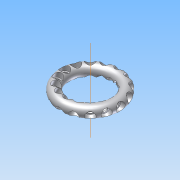
# Autodesk Inventor part: wheel
Saved by Autodesk Inventor 2012 (Build 160160000, 160)
## iProperties
Created: 2020-01-11
Part Number: wheel
Material: Default
Document SubType Name: Modeling
Designer: windows
Density: 1 g/cm^3
Mass: 34.9295 g
Surface Area: 256.992 cm^2
Volume: 34.9295 cm^3
Author: windows
Autodesk Inventor part; units mm, degrees
sketch "basic-frame" plane through (0, 0, 0) normal (0, 0, 1) x (1, 0, 0)
  line L0 (44.492, -8.85) -> (37.7185, -25.2027)
  line L1 (37.7185, -25.2027) -> (25.2027, -37.7185)
  line L2 (25.2027, -37.7185) -> (8.85, -44.492)
  line L3 (8.85, -44.492) -> (-8.85, -44.492)
  line L4 (-8.85, -44.492) -> (-25.2027, -37.7185)
  line L5 (-25.2027, -37.7185) -> (-37.7185, -25.2027)
  line L6 (-37.7185, -25.2027) -> (-44.492, -8.85)
  line L7 (-44.492, -8.85) -> (-44.492, 8.85)
  line L8 (-44.492, 8.85) -> (-37.7185, 25.2027)
  line L9 (-37.7185, 25.2027) -> (-25.2027, 37.7185)
  line L10 (-25.2027, 37.7185) -> (-8.85, 44.492)
  line L11 (-8.85, 44.492) -> (8.85, 44.492)
  line L12 (8.85, 44.492) -> (25.2027, 37.7185)
  line L13 (25.2027, 37.7185) -> (37.7185, 25.2027)
  line L14 (37.7185, 25.2027) -> (44.492, 8.85)
  line L15 (-73.9845, 0) -> (73.9845, 0) projected
  line L16 (44.492, 8.85) -> (44.492, -8.85)
  circle A0 centre (-44.492, 0) radius 7.6 construction
  circle A1 centre (-41.1052, -17.0263) radius 7.6 construction
  circle A2 centre (-31.4606, -31.4606) radius 7.6 construction
  circle A3 centre (-17.0263, -41.1052) radius 7.6 construction
  circle A4 centre (0, -44.492) radius 7.6 construction
  circle A5 centre (17.0263, -41.1052) radius 7.6 construction
  circle A6 centre (31.4606, -31.4606) radius 7.6 construction
  circle A7 centre (41.1052, -17.0263) radius 7.6 construction
  circle A8 centre (44.492, 0) radius 7.6 construction
  circle A9 centre (41.1052, 17.0263) radius 7.6 construction
  circle A10 centre (31.4606, 31.4606) radius 7.6 construction
  circle A11 centre (17.0263, 41.1052) radius 7.6 construction
  circle A12 centre (0, 44.492) radius 7.6 construction
  circle A13 centre (-17.0263, 41.1052) radius 7.6 construction
  circle A14 centre (-31.4606, 31.4606) radius 7.6 construction
  circle A15 centre (-41.1052, 17.0263) radius 7.6 construction
  circle A16 centre (-31.4606, 31.4606) radius 9.7599
  line L17 (-25.1935, 23.9786) -> (-37.7276, 38.9425)
  point P0 (0, 0)
  point P1 (0, 0)
  dimension "model_size" = 17.7
  dimension "d1" = 90.7272
  dimension "d106" = 15.2
  dimension "d109" = 360
  constraints: 34 end point, 17 centre point, 2 coincident, 2 midpoint, 2 point on circle, 2 point on line, 1 perpendicular, 1 tangent, 64 other
  measures "model_size" distance of L6.end L7.end
  measures "d1" distance of L0.start L7.end
  measures "d106" diameter of A0
ref_plane "plane-0" through (-44.492, -8.85, 0) normal (0, 0, 1) x (0, 1, 0)
sketch "circle-0" plane through (-44.492, -8.85, 0) normal (0, 0, 1) x (0, 1, 0)
  circle A0 centre (8.85, 0) radius 8.85
  line L0 (0, 0) -> (17.7, 0) projected
  circle A1 centre (8.85, 0) radius 7.6
  circle A2 centre (8.85, 0) radius 5
  point P0 (8.85, -44.492)
  dimension "model_de" = 15.2
  dimension "model_di" = 10
  constraints: 3 centre point, 2 coincident, 2 point on circle, 1 midpoint
  measures "model_de" diameter of A1
  measures "model_di" diameter of A2
ref_plane "plane-1" through (-37.7185, -25.2027, 0) normal (0.1802, 0.0747, 0.9808) x (-0.3827, 0.9239, 0)
sketch "circle-1" plane through (-37.7185, -25.2027, 0) normal (0.1802, 0.0747, 0.9808) x (-0.3827, 0.9239, 0)
  circle A0 centre (8.85, 0) radius 8.85
  line L0 (0, 0) -> (17.7, 0) projected
  circle A1 centre (8.85, 0) radius 5
  circle A2 centre (8.85, 0) radius 7.6
  point P0 (8.85, -43.6371)
  dimension "d76" = 10
  dimension "d77" = 15.2
  constraints: 3 centre point, 2 coincident, 2 point on circle, 1 midpoint
  measures "d76" diameter of A1
  measures "d77" diameter of A2
ref_plane "plane-2" through (-25.2027, -37.7185, 0) normal (0.2706, 0.2706, 0.9239) x (-0.7071, 0.7071, 0)
sketch "circle-2" plane through (-25.2027, -37.7185, 0) normal (0.2706, 0.2706, 0.9239) x (-0.7071, 0.7071, 0)
  line L0 (0, 0) -> (17.7, 0) projected
  circle A0 centre (8.85, 0) radius 8.85
  circle A1 centre (8.85, 0) radius 7.6
  circle A2 centre (8.85, 0) radius 5
  point P0 (8.85, -41.1052)
  dimension "d78" = 15.2
  dimension "d79" = 10
  constraints: 3 centre point, 2 coincident, 2 point on circle, 1 midpoint
  measures "d78" diameter of A1
  measures "d79" diameter of A2
ref_plane "plane-3" through (-8.85, -44.492, 0) normal (0.2126, 0.5133, 0.8315) x (-0.9239, 0.3827, 0)
sketch "circle-3" plane through (-8.85, -44.492, 0) normal (0.2126, 0.5133, 0.8315) x (-0.9239, 0.3827, 0)
  line L0 (0, 0) -> (17.7, 0) projected
  circle A0 centre (8.85, 0) radius 8.85
  circle A1 centre (8.85, 0) radius 7.6
  circle A2 centre (8.85, 0) radius 5
  point P0 (8.85, -36.9937)
  dimension "d80" = 15.2
  dimension "d81" = 10
  constraints: 3 coincident, 2 centre point, 1 horizontal alignment, 1 midpoint, 2 other
  measures "d80" diameter of A1
  measures "d81" diameter of A2
ref_plane "plane-4" through (8.85, -44.492, 0) normal (0, 0.7071, 0.7071) x (-1, 0, 0)
sketch "circle-4" plane through (8.85, -44.492, 0) normal (0, 0.7071, 0.7071) x (-1, 0, 0)
  circle A0 centre (8.85, 0) radius 8.85
  line L0 (0, 0) -> (17.7, 0) projected
  circle A1 centre (8.85, 0) radius 5
  circle A2 centre (8.85, 0) radius 7.6
  point P0 (8.85, -31.4606)
  dimension "d82" = 10
  dimension "d83" = 15.2
  constraints: 3 centre point, 2 coincident, 2 point on circle, 1 midpoint
  measures "d82" diameter of A1
  measures "d83" diameter of A2
ref_plane "plane-5" through (25.2027, -37.7185, 0) normal (-0.3182, 0.7682, 0.5556) x (-0.9239, -0.3827, 0)
sketch "circle-5" plane through (25.2027, -37.7185, 0) normal (-0.3182, 0.7682, 0.5556) x (-0.9239, -0.3827, 0)
  line L0 (0, 0) -> (17.7, 0) projected
  circle A0 centre (8.85, 0) radius 8.85
  circle A1 centre (8.85, 0) radius 7.6
  circle A2 centre (8.85, 0) radius 5
  point P0 (8.85, -24.7184)
  dimension "d84" = 15.2
  dimension "d85" = 10
  constraints: 3 centre point, 2 coincident, 2 point on circle, 1 midpoint
  measures "d84" diameter of A1
  measures "d85" diameter of A2
ref_plane "plane-6" through (37.7185, -25.2027, 0) normal (-0.6533, 0.6533, 0.3827) x (-0.7071, -0.7071, 0)
sketch "circle-6" plane through (37.7185, -25.2027, 0) normal (-0.6533, 0.6533, 0.3827) x (-0.7071, -0.7071, 0)
  circle A0 centre (8.85, 0) radius 8.85
  line L0 (0, 0) -> (17.7, 0) projected
  circle A1 centre (8.85, 0) radius 7.6
  circle A2 centre (8.85, 0) radius 5
  point P0 (8.85, -17.0263)
  dimension "d86" = 15.2
  dimension "d87" = 10
  constraints: 3 centre point, 2 coincident, 2 point on circle, 1 midpoint
  measures "d86" diameter of A1
  measures "d87" diameter of A2
ref_plane "plane-7" through (44.492, -8.85, 0) normal (-0.9061, 0.3753, 0.1951) x (-0.3827, -0.9239, 0)
sketch "circle-7" plane through (44.492, -8.85, 0) normal (-0.9061, 0.3753, 0.1951) x (-0.3827, -0.9239, 0)
  line L0 (0, 0) -> (17.7, 0) projected
  circle A0 centre (8.85, 0) radius 8.85
  circle A1 centre (8.85, 0) radius 7.6
  circle A2 centre (8.85, 0) radius 5
  point P0 (8.85, -8.6799)
  dimension "d88" = 15.2
  dimension "d89" = 10
  constraints: 3 centre point, 2 coincident, 2 point on circle, 1 midpoint
  measures "d88" diameter of A1
  measures "d89" diameter of A2
ref_plane "plane-8" through (44.492, 8.85, 0) normal (-1, 0, 0) x (0, -1, 0)
sketch "circle-8" plane through (44.492, 8.85, 0) normal (-1, 0, 0) x (0, -1, 0)
  circle A0 centre (8.85, 0) radius 8.85
  line L0 (0, 0) -> (17.7, 0) projected
  circle A1 centre (8.85, 0) radius 7.6
  circle A2 centre (8.85, 0) radius 5
  point P0 (8.85, 0)
  dimension "d90" = 15.2
  dimension "d91" = 10
  constraints: 3 centre point, 2 coincident, 2 point on circle, 1 midpoint
  measures "d90" diameter of A1
  measures "d91" diameter of A2
ref_plane "plane-9" through (37.7185, 25.2027, 0) normal (-0.9061, -0.3753, -0.1951) x (0.3827, -0.9239, 0)
sketch "circle-9" plane through (37.7185, 25.2027, 0) normal (-0.9061, -0.3753, -0.1951) x (0.3827, -0.9239, 0)
  circle A0 centre (8.85, 0) radius 8.85
  line L0 (0, 0) -> (17.7, 0) projected
  circle A1 centre (8.85, 0) radius 7.6
  circle A2 centre (8.85, 0) radius 5
  point P0 (8.85, 8.6799)
  dimension "d92" = 15.2
  dimension "d93" = 10
  constraints: 3 centre point, 2 coincident, 2 point on circle, 1 midpoint
  measures "d92" diameter of A1
  measures "d93" diameter of A2
ref_plane "plane-10" through (25.2027, 37.7185, 0) normal (-0.6533, -0.6533, -0.3827) x (0.7071, -0.7071, 0)
sketch "circle-10" plane through (25.2027, 37.7185, 0) normal (-0.6533, -0.6533, -0.3827) x (0.7071, -0.7071, 0)
  circle A0 centre (8.85, 0) radius 8.85
  line L0 (0, 0) -> (17.7, 0) projected
  circle A1 centre (8.85, 0) radius 7.6
  circle A2 centre (8.85, 0) radius 5
  point P0 (8.85, 17.0263)
  dimension "d94" = 15.2
  dimension "d95" = 10
  constraints: 3 centre point, 2 coincident, 2 point on circle, 1 midpoint
  measures "d94" diameter of A1
  measures "d95" diameter of A2
ref_plane "plane-11" through (8.85, 44.492, 0) normal (-0.3182, -0.7682, -0.5556) x (0.9239, -0.3827, 0)
sketch "circle-11" plane through (8.85, 44.492, 0) normal (-0.3182, -0.7682, -0.5556) x (0.9239, -0.3827, 0)
  circle A0 centre (8.85, 0) radius 8.85
  line L0 (0, 0) -> (17.7, 0) projected
  circle A1 centre (8.85, 0) radius 7.6
  circle A2 centre (8.85, 0) radius 5
  point P0 (8.85, 24.7184)
  dimension "d96" = 15.2
  dimension "d97" = 10
  constraints: 3 centre point, 2 coincident, 2 point on circle, 1 midpoint
  measures "d96" diameter of A1
  measures "d97" diameter of A2
ref_plane "plane-12" through (-8.85, 44.492, 0) normal (0, -0.7071, -0.7071) x (1, 0, 0)
sketch "circle-12" plane through (-8.85, 44.492, 0) normal (0, -0.7071, -0.7071) x (1, 0, 0)
  circle A0 centre (8.85, 0) radius 8.85
  line L0 (0, 0) -> (17.7, 0) projected
  circle A1 centre (8.85, 0) radius 7.6
  circle A2 centre (8.85, 0) radius 5
  point P0 (8.85, 31.4606)
  dimension "d98" = 15.2
  dimension "d99" = 10
  constraints: 3 centre point, 2 coincident, 2 point on circle, 1 midpoint
  measures "d98" diameter of A1
  measures "d99" diameter of A2
ref_plane "plane-13" through (-25.2027, 37.7185, 0) normal (0.2126, -0.5133, -0.8315) x (0.9239, 0.3827, 0)
sketch "circle-13" plane through (-25.2027, 37.7185, 0) normal (0.2126, -0.5133, -0.8315) x (0.9239, 0.3827, 0)
  circle A0 centre (8.85, 0) radius 8.85
  line L0 (0, 0) -> (17.7, 0) projected
  circle A1 centre (8.85, 0) radius 7.6
  circle A2 centre (8.85, 0) radius 5
  point P0 (8.85, 36.9937)
  dimension "d100" = 15.2
  dimension "d101" = 10
  constraints: 3 centre point, 2 coincident, 2 point on circle, 1 midpoint
  measures "d100" diameter of A1
  measures "d101" diameter of A2
ref_plane "plane-14" through (-37.7185, 25.2027, 0) normal (0.2706, -0.2706, -0.9239) x (0.7071, 0.7071, 0)
sketch "circle-14" plane through (-37.7185, 25.2027, 0) normal (0.2706, -0.2706, -0.9239) x (0.7071, 0.7071, 0)
  circle A0 centre (8.85, 0) radius 8.85
  line L0 (0, 0) -> (17.7, 0) projected
  circle A1 centre (8.85, 0) radius 7.6
  circle A2 centre (8.85, 0) radius 5
  point P0 (8.85, 41.1052)
  dimension "d102" = 15.2
  dimension "d103" = 10
  constraints: 3 centre point, 2 coincident, 2 point on circle, 1 midpoint
  measures "d102" diameter of A1
  measures "d103" diameter of A2
ref_plane "plane-15" through (-44.492, 8.85, 0) normal (0.1802, -0.0747, -0.9808) x (0.3827, 0.9239, 0)
sketch "circle-15" plane through (-44.492, 8.85, 0) normal (0.1802, -0.0747, -0.9808) x (0.3827, 0.9239, 0)
  line L0 (0, 0) -> (17.7, 0) projected
  circle A0 centre (8.85, 0) radius 8.85
  circle A1 centre (8.85, 0) radius 7.6
  circle A2 centre (8.85, 0) radius 5
  point P0 (8.85, 43.6371)
  dimension "d104" = 15.2
  dimension "d105" = 10
  constraints: 3 centre point, 2 coincident, 2 point on circle, 1 midpoint
  measures "d104" diameter of A1
  measures "d105" diameter of A2
ref_plane "工作平面17" through (-31.4606, 31.4606, 0) normal (0, 0, 1) x (1, 0, 0)
ref_plane "工作平面18" through (-31.4606, 31.4606, 0) normal (0.7071, 0.7071, 0) x (0, 0, 1)
sketch "草图22" plane through (-31.4606, 31.4606, 0) normal (0.7071, 0.7071, 0) x (0, 0, 1)
  line L0 (0, -9.7599) -> (0, 9.7599) projected
  line L1 (-14.0758, 0) -> (14.0758, 0) projected
  circle A0 centre (0, 0) radius 9.7599
  line L2 (-14.0758, 44.492) -> (14.0758, 44.492) projected
  point P0 (0, 44.492)
  constraints: 2 midpoint, 1 vertical alignment, 2 other
revolve "tire" add sketch "草图22" angle 360 about axis through (0, 0, -10) along (0, 0, 1)
extrude "hole0" cut sketch "circle-0" along normal through all both and the other way through all contours A1 L0 A2 | L0 A2 A1 | A2 L0 | L0 A2
extrude "support0" add sketch "circle-0" along normal mid plane 2 contours A1 L0 A2 | L0 A2 A1
extrude "hole1" cut sketch "circle-1" along normal through all both and the other way through all contours A2 L0 A1 | L0 A1 A2 | A1 L0 | L0 A1
extrude "support1" add sketch "circle-1" along normal mid plane 2 contours A2 L0 A1 | L0 A1 A2
extrude "hole2" cut sketch "circle-2" along normal through all both and the other way through all contours A2 L0 A1 | A2 L0 | L0 A2 | L0 A1 A2
extrude "support2" add sketch "circle-2" along normal mid plane 2 contours A2 L0 A1 | L0 A1 A2
extrude "hole3" cut sketch "circle-3" along normal through all both and the other way through all contours A2 L0 A1 | A2 L0 | L0 A2 | L0 A1 A2
extrude "support3" add sketch "circle-3" along normal mid plane 2 contours A2 L0 A1 | L0 A1 A2
extrude "hole4" cut sketch "circle-4" along normal through all both and the other way through all contours A2 L0 A1 | L0 A1 A2 | A1 L0 | L0 A1
extrude "support4" add sketch "circle-4" along normal mid plane 2 contours A2 L0 A1 | L0 A1 A2
extrude "hole5" cut sketch "circle-5" along normal through all both and the other way through all contours A2 L0 A1 | A2 L0 | L0 A2 | L0 A1 A2
extrude "support5" add sketch "circle-5" along normal mid plane 2 contours A2 L0 A1 | L0 A1 A2
extrude "hole6" cut sketch "circle-6" along normal through all both and the other way through all contours A1 L0 A2 | L0 A2 A1 | A2 L0 | L0 A2
extrude "support6" add sketch "circle-6" along normal mid plane 2 contours A1 L0 A2 | L0 A2 A1
extrude "hole7" cut sketch "circle-7" along normal through all both and the other way through all contours A2 L0 A1 | A2 L0 | L0 A2 | L0 A1 A2
extrude "support7" add sketch "circle-7" along normal mid plane 2 contours A2 L0 A1 | L0 A1 A2
extrude "hole8" cut sketch "circle-8" along normal mid plane 35.4 contours A1 L0 A2 | L0 A2 A1 | A2 L0 | L0 A2
extrude "support8" add sketch "circle-8" along normal mid plane 2 contours A1 L0 A2 | L0 A2 A1
extrude "hole9" cut sketch "circle-9" along normal through all both and the other way through all contours A1 L0 A2 | L0 A2 A1 | A2 L0 | L0 A2
extrude "support9" add sketch "circle-9" along normal mid plane 2 contours A1 L0 A2 | L0 A2 A1
extrude "hole10" cut sketch "circle-10" along normal through all both and the other way through all contours A1 L0 A2 | L0 A2 A1 | A2 L0 | L0 A2
extrude "support10" add sketch "circle-10" along normal mid plane 2 contours A1 L0 A2 | L0 A2 A1
extrude "hole11" cut sketch "circle-11" along normal through all both and the other way through all contours A1 L0 A2 | L0 A2 A1 | A2 L0 | L0 A2
extrude "support11" add sketch "circle-11" along normal mid plane 2 contours A1 L0 A2 | L0 A2 A1
extrude "hole12" cut sketch "circle-12" along normal through all both and the other way through all contours A1 L0 A2 | L0 A2 A1 | A2 L0 | L0 A2
extrude "support12" add sketch "circle-12" along normal mid plane 2 contours A1 L0 A2 | L0 A2 A1
extrude "hole13" cut sketch "circle-13" along normal through all both and the other way through all contours A1 L0 A2 | L0 A2 A1 | A2 L0 | L0 A2
extrude "support13" add sketch "circle-13" along normal mid plane 2 contours A1 L0 A2 | L0 A2 A1
extrude "hole14" cut sketch "circle-14" along normal through all both and the other way through all contours A1 L0 A2 | L0 A2 A1 | A2 L0 | L0 A2
extrude "support14" add sketch "circle-14" along normal mid plane 2 contours A1 L0 A2 | L0 A2 A1
extrude "hole15" cut sketch "circle-15" along normal through all both and the other way through all contours A2 L0 A1 | A2 L0 | L0 A2 | L0 A1 A2
extrude "support15" add sketch "circle-15" along normal mid plane 2 contours A2 L0 A1 | L0 A1 A2
equation "\"model_size\" = size"
equation "\"d106\" = model_de"
equation "\"model_de\" = de"
equation "\"model_di\" = di"
equation "\"d76\" = model_di"
equation "\"d77\" = model_de"
equation "\"d78\" = model_de"
equation "\"d79\" = model_di"
equation "\"d80\" = model_de"
equation "\"d81\" = model_di"
equation "\"d82\" = model_di"
equation "\"d83\" = model_de"
equation "\"d84\" = model_de"
equation "\"d85\" = model_di"
equation "\"d86\" = model_de"
equation "\"d87\" = model_di"
equation "\"d88\" = model_de"
equation "\"d89\" = model_di"
equation "\"d90\" = model_de"
equation "\"d91\" = model_di"
equation "\"d92\" = model_de"
equation "\"d93\" = model_di"
equation "\"d94\" = model_de"
equation "\"d95\" = model_di"
equation "\"d96\" = model_de"
equation "\"d97\" = model_di"
equation "\"d98\" = model_de"
equation "\"d99\" = model_di"
equation "\"d100\" = model_de"
equation "\"d101\" = model_di"
equation "\"d102\" = model_de"
equation "\"d103\" = model_di"
equation "\"d104\" = model_de"
equation "\"d105\" = model_di"
equation "\"d121\" = model_thickness"
equation "\"d123\" = model_thickness"
equation "\"d125\" = model_thickness"
equation "\"d127\" = model_thickness"
equation "\"d129\" = model_thickness"
equation "\"d131\" = model_thickness"
equation "\"d133\" = model_thickness"
equation "\"d135\" = model_thickness"
equation "\"d137\" = model_thickness"
equation "\"d139\" = model_thickness"
equation "\"d141\" = model_thickness"
equation "\"d143\" = model_thickness"
equation "\"d145\" = model_thickness"
equation "\"d147\" = model_thickness"
equation "\"d149\" = model_thickness"
equation "\"d151\" = 2 * model_size"
equation "\"d153\" = model_thickness"
equation "\"d155\" = model_thickness"
equation "\"d157\" = model_thickness"
equation "\"d159\" = model_thickness"
equation "\"d161\" = model_thickness"
equation "\"d163\" = model_thickness"
equation "\"d165\" = model_thickness"
equation "\"d168\" = model_thickness"
equation "\"d170\" = model_thickness"
equation "\"d172\" = model_thickness"
equation "\"d174\" = model_thickness"
equation "\"d176\" = model_thickness"
equation "\"d178\" = model_thickness"
equation "\"d115\" = model_size"
equation "\"model_thickness\" = thickness"
equation "\"d14\" = rotation"
equation "\"d15\" = 2 * rotation"
equation "\"d16\" = 3 * rotation"
equation "\"d17\" = 4 * rotation"
equation "\"d18\" = 5 * rotation"
equation "\"d19\" = 6 * rotation"
equation "\"d20\" = 7 * rotation"
equation "\"d21\" = 8 * rotation"
equation "\"d22\" = 9 * rotation"
equation "\"d23\" = 10 * rotation"
equation "\"d24\" = 11 * rotation"
equation "\"d25\" = 12 * rotation"
equation "\"d26\" = 13 * rotation"
equation "\"d27\" = 14 * rotation"
equation "\"d28\" = 15 * rotation"
equation "\"size\" = 17.7"
equation "\"de\" = 15.2"
equation "\"di\" = 10"
equation "\"thickness\" = 2"
